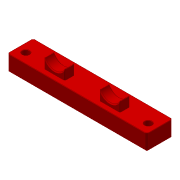
# Autodesk Inventor part: single extruder securer
Saved by Autodesk Inventor 2015 (Build 190159000, 159)
## iProperties
Created: 2020-04-10
Part Number: single extruder securer
Material: Generic
Document SubType Name: Modeling
Designer: Ghassan Yusuf
Density: 1 g/cm^3
Appearance: Default(1)
Author: Ghassan Yusuf
Autodesk Inventor part; units mm, degrees
ref_plane "YZ Plane" through (0, 0, 0) normal (1, 0, 0) x (0, 1, 0)
ref_plane "XZ Plane" through (0, 0, 0) normal (0, 1, 0) x (-1, 0, 0)
ref_plane "XY Plane" through (0, 0, 0) normal (0, 0, 1) x (1, 0, 0)
sketch "Sketch1" plane through (0, 0, 0) normal (0, 0, 1) x (1, 0, 0)
  line L0 (-40.5, 7.5) -> (40.5, 7.5)
  line L1 (40.5, 7.5) -> (40.5, -7.5)
  line L2 (40.5, -7.5) -> (-40.5, -7.5)
  line L3 (-40.5, -7.5) -> (-40.5, 7.5)
  circle A0 centre (-35.5, -1.7) radius 2
  circle A1 centre (35.5, -1.7) radius 2
  point P0 (0, 0)
  point P1 (-40.5, 0)
  point P2 (0, 7.5)
  dimension "d0" = 81
  dimension "d1" = 15
  dimension "d2" = 4
  dimension "d7" = 9.2
  dimension "d8" = 9.2
  dimension "d41" = 5
  dimension "d42" = 5
  constraints: 8 end point, 2 centre point, 2 horizontal alignment, 2 midpoint, 2 parallel, 1 equal radius, 1 horizontal, 1 perpendicular, 1 vertical alignment
  measures "d0" distance of L1.end L2.end
  measures "d1" distance of L0.end L1.end
  measures "d2" diameter of A0
  measures "d7" distance from line of L0 A0.centre
  measures "d8" distance from line of A1.centre L0
  measures "d41" distance from line of A0.centre L3
  measures "d42" distance from line of L1 A1.centre
extrude "Extrusion1" add sketch "Sketch1" along normal mid plane 9.5
sketch "Sketch2" plane through (0, 0, 4.75) normal (0, 0, 1) x (1, 0, 0)
  line L0 (9.85, 1.2) -> (22.15, 1.2)
  line L1 (22.15, 1.2) -> (22.15, -4.6)
  line L2 (22.15, -4.6) -> (9.85, -4.6)
  line L3 (9.85, -4.6) -> (9.85, 1.2)
  line L4 (-40.5, 7.5) -> (40.5, 7.5) projected
  line L5 (40.5, -7.5) -> (40.5, 7.5) projected
  line L6 (10, 1.2) -> (10, -4.6)
  line L7 (-40.5, -7.5) -> (40.5, -7.5) projected
  line L8 (22, 1.2) -> (22, -4.6)
  line L9 (16, 1.2) -> (16, -4.6)
  line L10 (-9.85, 1.2) -> (-22.15, 1.2)
  line L11 (-22.15, 1.2) -> (-22.15, -4.6)
  line L12 (-22.15, -4.6) -> (-9.85, -4.6)
  line L13 (-9.85, -4.6) -> (-9.85, 1.2)
  line L14 (-16, 1.2) -> (-16, -4.6)
  line L15 (-40.5, 7.5) -> (-40.5, -7.5) projected
  line L16 (-22, 1.2) -> (-22, -4.6)
  line L17 (-10, 1.2) -> (-10, -4.6)
  point P0 (0, 0)
  dimension "d10" = 5.8
  dimension "d11" = 6.3
  dimension "d12" = 12.3
  dimension "d14" = 0.15
  dimension "d43" = 24.5
  dimension "d44" = 24.5
  dimension "d45" = 0.15
  dimension "d46" = 0.15
  constraints: 28 end point, 8 point on line, 5 parallel, 4 midpoint, 3 collinear, 3 perpendicular, 2 horizontal, 2 vertical
  measures "d10" distance of L0.end L1.end
  measures "d11" distance between parallel lines of L4 L0
  measures "d12" distance between parallel lines of L1 L3
  measures "d14" distance between parallel lines of L3 L6
  measures "d43" distance between parallel lines of L5 L9
  measures "d44" distance between parallel lines of L15 L14
  measures "d45" distance between parallel lines of L11 L16
  measures "d46" distance between parallel lines of L13 L17
extrude "Extrusion3" add sketch "Sketch2" along normal blind 8 contours L0 L9 L2 L6 | L0 L8 L2 L9 | L17 L12 L14 L10 | L14 L12 L16 L10
sketch "Sketch3" plane through (10, 1.2, 4.75) normal (0, 1, 0) x (1, 0, 0)
  line L0 (0, -8) -> (12, -8) projected
  circle A0 centre (6, -8) radius 6.15
  line L1 (-20, -8) -> (-32, -8) projected
  circle A1 centre (-26, -8) radius 6.15
  point P0 (-10, 4.75)
  dimension "d20" = 12.3
  constraints: 2 centre point, 2 midpoint, 1 equal radius
  measures "d20" diameter of A0
extrude "Extrusion4" cut sketch "Sketch3" against normal blind 8
chamfer "Chamfer1" distance 0.5 angle 45 8 edges at (10, -4.6, 8.075) (10, 1.2, 8.075) (22, 1.2, 8.075) (22, -4.6, 8.075) (-10, -4.6, 8.075) (-10, 1.2, 8.075) (-22, -4.6, 8.075) (-22, 1.2, 8.075)
chamfer "Chamfer2" distance 0.5 angle 45 4 edges at (16, -4.6, 6.6) (16, 1.2, 6.6) (-16, -4.6, 6.6) (-16, 1.2, 6.6)
fillet "Fillet1" radius 0.2 4 edges at (10, -1.7, 11.4) (22, -1.7, 11.4) (-22, -1.7, 11.4) (-10, -1.7, 11.4)
chamfer "Chamfer3" distance 1 angle 45 8 edges at (40.5, 0, -4.75) (-40.5, 0, -4.75) (0, 7.5, -4.75) (40.5, 7.5, 0) (-40.5, 7.5, 0) (40.5, -7.5, 0) (0, -7.5, -4.75) (-40.5, -7.5, 0)
sketch "Sketch4" plane through (0, 0, -4.75) normal (0, 0, -1) x (-1, 0, 0)
  circle A0 centre (-35.5, -1.7) radius 2 projected
  circle A1 centre (-35.5, -1.7) radius 3
  circle A2 centre (35.5, -1.7) radius 2 projected
  circle A3 centre (35.5, -1.7) radius 3
  point P0 (0, 0)
  dimension "d33" = 6
  dimension "d34" = 6
  constraints: 2 centre point, 2 coincident
  measures "d33" diameter of A1
  measures "d34" diameter of A3
extrude "Extrusion5" cut sketch "Sketch4" against normal blind 3 contours A0 | A1 | A2 | A3
fillet "Fillet2" radius 0.2 8 edges at (0, 7.5, 4.75) (0, -7.5, 4.75) (-40.5, 0, 4.75) (40.5, 0, 4.75) (40, 7, 4.75) (40, -7, 4.75) (-40, -7, 4.75) (-40, 7, 4.75)
chamfer "Chamfer4" distance 0.2 angle 45 4 edges at (-37.5, -1.7, 4.75) (33.5, -1.7, 4.75) (-37.5, -1.7, -1.75) (33.5, -1.7, -1.75)
sketch "Sketch5" plane through (0, 0, -4.75) normal (0, 0, -1) x (-1, 0, 0)
  line L0 (-40.5, 7.5) -> (40.5, 7.5) construction
  line L1 (40.5, 7.5) -> (40.5, -7.5) construction
  line L2 (40.5, -7.5) -> (-40.5, -7.5) construction
  line L3 (-40.5, -7.5) -> (-40.5, 7.5) construction
  line L4 (39.5, 7.5) -> (-39.5, 7.5) projected
  line L5 (-40.5, 6.5) -> (-40.5, -6.5) projected
  line L6 (-29.8055, -5) -> (-29.8055, 3.0956)
  line L7 (-29.8055, 3.0956) -> (-32.7634, 3.0956)
  line L8 (-32.7634, 3.0956) -> (-32.7634, 5)
  line L9 (-32.7634, 5) -> (-24.3355, 5)
  line L10 (-24.3355, 5) -> (-24.3355, 3.0956)
  line L11 (-24.3355, 3.0956) -> (-27.2934, 3.0956)
  line L12 (-27.2934, 3.0956) -> (-27.2934, -5)
  line L13 (-27.2934, -5) -> (-29.8055, -5)
  line L14 (-24.3841, -5) -> (-21.0049, 5)
  line L15 (-21.0049, 5) -> (-18.2658, 5)
  line L16 (-18.2658, 5) -> (-14.8865, -5)
  line L17 (-14.8865, -5) -> (-17.4716, -5)
  line L18 (-17.4716, -5) -> (-18.0956, -2.9579)
  line L19 (-18.0956, -2.9579) -> (-21.2399, -2.9579)
  line L20 (-21.2399, -2.9579) -> (-21.872, -5)
  line L21 (-21.872, -5) -> (-24.3841, -5)
  line L22 (-18.6467, -1.1426) -> (-19.6677, 2.1637)
  line L23 (-19.6677, 2.1637) -> (-20.6969, -1.1426)
  line L24 (-20.6969, -1.1426) -> (-18.6467, -1.1426)
  line L25 (-5.1297, -5) -> (-8.1686, -5)
  line L26 (-8.1686, -5) -> (-10.8833, -0.94)
  line L27 (-10.8833, -0.94) -> (-11.3776, -1.6207)
  line L28 (-11.3776, -1.6207) -> (-11.3776, -5)
  line L29 (-11.3776, -5) -> (-13.8898, -5)
  line L30 (-13.8898, -5) -> (-13.8898, 5)
  line L31 (-13.8898, 5) -> (-11.3776, 5)
  line L32 (-11.3776, 5) -> (-11.3776, 0.5348)
  line L33 (-11.3776, 0.5348) -> (-8.1686, 5)
  line L34 (-8.1686, 5) -> (-5.2755, 5)
  line L35 (-5.2755, 5) -> (-8.8412, 0.3566)
  line L36 (-8.8412, 0.3566) -> (-5.1297, -5)
  line L37 (-4.3112, -5) -> (-4.3112, 5)
  line L38 (-4.3112, 5) -> (2.4473, 5)
  line L39 (2.4473, 5) -> (2.4473, 3.0956)
  line L40 (2.4473, 3.0956) -> (-1.8152, 3.0956)
  line L41 (-1.8152, 3.0956) -> (-1.8152, 1.3371)
  line L42 (-1.8152, 1.3371) -> (2.1151, 1.3371)
  line L43 (2.1151, 1.3371) -> (2.1151, -0.5673)
  line L44 (2.1151, -0.5673) -> (-1.8152, -0.5673)
  line L45 (-1.8152, -0.5673) -> (-1.8152, -3.0956)
  line L46 (-1.8152, -3.0956) -> (2.4473, -3.0956)
  line L47 (2.4473, -3.0956) -> (2.4473, -5)
  line L48 (2.4473, -5) -> (-4.3112, -5)
  spline S0 degree 2 poles (13.2496, 0) (13.2496, -2.4311) (10.6564, -5.2107) (8.4036, -5.2107) knots 0 0 0 1 2 2 2
  spline S1 degree 2 poles (8.4036, -5.2107) (6.1426, -5.2107) (3.5656, -2.3987) (3.5656, 0) knots 0 0 0 1 2 2 2
  spline S2 degree 2 poles (3.5656, 0) (3.5656, 2.4068) (6.1426, 5.2107) (8.4036, 5.2107) knots 0 0 0 1 2 2 2
  spline S3 degree 2 poles (8.4036, 5.2107) (10.6564, 5.2107) (13.2496, 2.423) (13.2496, 0) knots 0 0 0 1 2 2 2
  spline S4 degree 2 poles (10.6564, 0) (10.6564, 0.8995) (10.2917, 2.1556) (9.9757, 2.5527) knots 0 0 0 1 2 2 2
  spline S5 degree 2 poles (9.9757, 2.5527) (9.6596, 2.966) (8.8493, 3.3225) (8.4117, 3.3225) knots 0 0 0 1 2 2 2
  spline S6 degree 2 poles (8.4117, 3.3225) (7.9498, 3.3225) (7.1961, 2.9903) (6.8476, 2.5689) knots 0 0 0 1 2 2 2
  spline S7 degree 2 poles (6.8476, 2.5689) (6.5397, 2.1799) (6.1588, 0.8914) (6.1588, 0) knots 0 0 0 1 2 2 2
  spline S8 degree 2 poles (6.1588, 0) (6.1588, -0.9238) (6.5235, -2.1394) (6.8395, -2.5527) knots 0 0 0 1 2 2 2
  spline S9 degree 2 poles (6.8395, -2.5527) (7.1556, -2.966) (7.9741, -3.3225) (8.4117, -3.3225) knots 0 0 0 1 2 2 2
  spline S10 degree 2 poles (8.4117, -3.3225) (8.8574, -3.3225) (9.684, -2.9417) (9.9838, -2.5365) knots 0 0 0 1 2 2 2
  spline S11 degree 2 poles (9.9838, -2.5365) (10.3079, -2.0989) (10.6564, -0.94) (10.6564, 0) knots 0 0 0 1 2 2 2
  line L49 (23.3063, -5) -> (20.8914, -5)
  line L50 (20.8914, -5) -> (17.034, 1.9692)
  line L51 (17.034, 1.9692) -> (17.034, -5)
  line L52 (17.034, -5) -> (14.7407, -5)
  line L53 (14.7407, -5) -> (14.7407, 5)
  line L54 (14.7407, 5) -> (17.8201, 5)
  line L55 (17.8201, 5) -> (21.013, -0.7293)
  line L56 (21.013, -0.7293) -> (21.013, 5)
  line L57 (21.013, 5) -> (23.3063, 5)
  line L58 (23.3063, 5) -> (23.3063, -5)
  line L59 (25.3404, -5) -> (25.3404, 5)
  line L60 (25.3404, 5) -> (32.0989, 5)
  line L61 (32.0989, 5) -> (32.0989, 3.0956)
  line L62 (32.0989, 3.0956) -> (27.8363, 3.0956)
  line L63 (27.8363, 3.0956) -> (27.8363, 1.3371)
  line L64 (27.8363, 1.3371) -> (31.7666, 1.3371)
  line L65 (31.7666, 1.3371) -> (31.7666, -0.5673)
  line L66 (31.7666, -0.5673) -> (27.8363, -0.5673)
  line L67 (27.8363, -0.5673) -> (27.8363, -3.0956)
  line L68 (27.8363, -3.0956) -> (32.0989, -3.0956)
  line L69 (32.0989, -3.0956) -> (32.0989, -5)
  line L70 (32.0989, -5) -> (25.3404, -5)
  point P0 (0, 0)
  point P1 (0, 7.5)
  point P2 (0, 7.5)
  point P3 (-40.5, 0)
  point P4 (-40.5, 0)
  constraints: 4 midpoint, 2 coincident, 2 collinear, 2 other
emboss "Emboss1" sketch "Sketch5" operation cut depth 1 direction (0, 0, 1)
equation "\"d42\" = d41"
equation "\"d44\" = d43"
equation "\"d46\" = d45"
body "Solid1"
